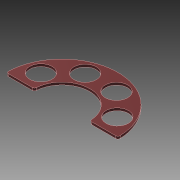
# Autodesk Inventor part: Фиксатор
Saved by Autodesk Inventor 2022 (Build 260153000, 153)
## iProperties
RuleStatus: InUse
Part Number: Фиксатор
Checked By: Якушев
Engr Approved By: Малов
Material: По умолчанию1
Document SubType Name: Modeling
Mfg Approved By: Судаков
Designer: Смирнов
Density: 1 g/cm^3
Appearance: Каштановый
AfterMaterialChange0: Материал
BeforeDocSave0: Материал
AfterAnyiPropertyChange0: Материал
Материал: По умолчанию1
Author: Смирнов
Autodesk Inventor part; units mm, degrees
ref_plane "YZ Plane" through (0, 0, 0) normal (1, 0, 0) x (0, 1, 0)
ref_plane "XZ Plane" through (0, 0, 0) normal (0, 1, 0) x (-1, 0, 0)
ref_plane "РабПлоскость1" through (0, 0, 3) normal (0, 0, 1) x (1, 0, 0)
sketch "Эскиз1" plane through (0, 0, 3) normal (0, 0, 1) x (1, 0, 0)
  circle A0 centre (0, 0) radius 135 projected
  circle A1 centre (0, 0) radius 101 construction
  line L0 (0, 0) -> (0, 184.3698) construction
  circle A2 centre (-37.8353, 93.6456) radius 27
  circle A3 centre (-92.2681, 41.0804) radius 27
  circle A4 centre (37.8353, 93.6456) radius 27
  circle A5 centre (92.2681, 41.0804) radius 27
  line L1 (0, 0) -> (37.8353, 93.6456) construction
  line L2 (0, 0) -> (92.2681, 41.0804) construction
  circle A6 centre (0, 0) radius 67
  line L3 (-135, 0) -> (135, 0)
  circle A7 centre (120, 0) radius 1.6 construction
  circle A8 centre (-120, 0) radius 1.6 construction
  circle A9 centre (120, 0) radius 8 construction
  circle A10 centre (-120, 0) radius 8 construction
  circle A11 centre (0, 120) radius 1.6 construction
  circle A12 centre (0, 120) radius 8 construction
  line L4 (0, 0) -> (-116.9134, -67.5) construction
  line L5 (0, 0) -> (116.9134, -67.5) construction
  point P0 (67, 0)
  point P1 (-67, 0)
  point P2 (-128, 0)
  point P3 (-112, 0)
  point P4 (112, 0)
  point P5 (128, 0)
  dimension "d0" = 54
  dimension "d3" = 202
  dimension "d4" = 34
  dimension "d5" = 34
  dimension "d9" = 16
  dimension "d11" = 120
  dimension "d12" = 22
  dimension "d13" = 44
  constraints: 12 end point, 9 centre point, 8 point on circle, 5 coincident, 3 equal radius, 1 horizontal, 1 midpoint, 1 vertical, 3 other
  measures "d0" diameter of A4
  measures "d3" diameter of A1
  measures "d4" radial gap between concentric circles of A0 A1
  measures "d5" radial gap between concentric circles of A6 A1
  measures "d9" diameter of A9
  measures "d11" angle of L5 L4
  measures "d12" angle of L1 L0
  measures "d13" angle of L2 L1
extrude "Выдавливание1" add sketch "Эскиз1" along normal blind 6 contours L3 A6 A0 picked at (99.1742, 4.7591)
fillet "Сопряжение1" radius 5 4 edges at (-67, 0, 6) (-135, 0, 6) (67, 0, 6) (135, 0, 6)
equation "\"d5\" = d4"
equation "\"d13\" = 2 * d12"
